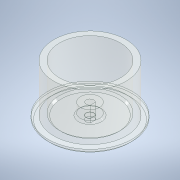
# Autodesk Inventor part: Kolo
Saved by Autodesk Inventor 2020 (Build 240168000, 168)
## iProperties
Created: 2020-02-11
Part Number: Kolo
Material: Glass
Document SubType Name: Modeling
Designer: atmat
Density: 2.18 g/cm^3
Appearance: Clear
Mass: 28.2894 g
Surface Area: 100.3 cm^2
Volume: 12.9768 cm^3
Author: atmat
Autodesk Inventor part; units mm, degrees
ref_plane "YZ Plane" through (0, 0, 0) normal (1, 0, 0) x (0, 1, 0)
ref_plane "XZ Plane" through (0, 0, 0) normal (0, 1, 0) x (-1, 0, 0)
sketch "Sketch1" plane through (0, 0, 0) normal (0, 1, 0) x (-1, 0, 0)
  circle A0 centre (0, 0) radius 19
  circle A1 centre (0, 0) radius 16
  dimension "d0" = 38
  dimension "d1" = 3
  constraints: 2 centre point, 2 coincident
  measures "d0" diameter of A0
  measures "d1" radial gap between concentric circles of A0 A1
extrude "Extrusion1" add sketch "Sketch1" along normal blind 25
sketch "Sketch2" plane through (0, 0, 0) normal (0, -1, 0) x (1, 0, 0)
  circle A0 centre (0, 0) radius 22
  circle A1 centre (0, 0) radius 19 projected
  dimension "d4" = 3
  constraints: 1 centre point, 1 coincident
  measures "d4" radial gap between concentric circles of A0 A1
extrude "Extrusion2" add sketch "Sketch2" along normal blind 2 contours A0 | A1
ref_plane "Work Plane1" through (0, -2, 0) normal (0, -1, 0) x (1, 0, 0)
sketch "Sketch3" plane through (0, -2, 0) normal (0, -1, 0) x (1, 0, 0)
  circle A0 centre (0, 0) radius 2.125
  line L0 (1.625, -4.5) -> (1.625, 4.5)
  point P0 (1.625, -1.3693)
  point P1 (1.625, 1.3693)
  dimension "d8" = 4.25
  dimension "d9" = 9
  dimension "d10" = 4.5
  dimension "d11" = 1.625
  constraints: 2 end point, 1 centre point, 1 coincident, 1 vertical
  measures "d8" diameter of A0
  measures "d9" distance of L0.start L0.end
  measures "d10" vertical distance of point (0, 0) L0.start
  measures "d11" distance from line of point (0, 0) L0
extrude "Extrusion3" cut sketch "Sketch3" against normal blind 28 contours L0 A0 picked at (0.375, 0)
sketch "Sketch4" plane through (0, 0, 0) normal (0, 1, 0) x (1, 0, 0)
  circle A0 centre (0, 0) radius 5
  circle A1 centre (0, 0) radius 2
  line L0 (1.5, -1.3229) -> (1.5, 1.3229) projected
  line L1 (1.5, 1.3229) -> (1.5, -1.3229)
  dimension "d14" = 3
  dimension "d15" = 4
  constraints: 2 centre point, 2 coincident, 2 end point, 1 collinear
  measures "d14" radial gap between concentric circles of A1 A0
  measures "d15" diameter of A1
extrude "Extrusion4" add sketch "Sketch4" along normal blind 6 contours A0 | A1 L0 picked at (1.5908, -0.3089)
chamfer "Chamfer1" distance 1 angle 45 1 edges at (-22, -2, 0)
chamfer "Chamfer2" distance 1 angle 45 2 edges at (16, 0, 0) (-5, 0, 0)
body "Solid1"
